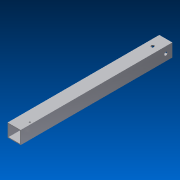
# Autodesk Inventor part: SwitchBarSupport
Saved by Autodesk Inventor 2013 (Build 170138000, 138)
## iProperties
Created: 2013-07-20
Part Number: SwitchBarSupport
Material: Aluminum 6061
Document SubType Name: Modeling
Designer: robotics
Density: 1 g/cm^3
Author: robotics
Autodesk Inventor part; units mm, degrees
ref_plane "YZ Plane" through (0, 0, 0) normal (1, 0, 0) x (0, 1, 0)
ref_plane "XZ Plane" through (0, 0, 0) normal (0, 1, 0) x (-1, 0, 0)
ref_plane "XY Plane" through (0, 0, 0) normal (0, 0, 1) x (1, 0, 0)
sketch "Sketch1" plane through (0, 0, 0) normal (0, 0, 1) x (1, 0, 0)
  line L0 (0, 0) -> (25.4, 0)
  line L1 (25.4, 0) -> (25.4, 25.4)
  line L2 (25.4, 25.4) -> (0, 25.4)
  line L3 (0, 25.4) -> (0, 0)
  line L4 (1.5875, 1.5875) -> (23.8125, 1.5875)
  line L5 (23.8125, 1.5875) -> (23.8125, 23.8125)
  line L6 (23.8125, 23.8125) -> (1.5875, 23.8125)
  line L7 (1.5875, 23.8125) -> (1.5875, 1.5875)
  dimension "d0" = 25.4
  dimension "d1" = 25.4
  dimension "d2" = 1.5875
  dimension "d3" = 1.5875
  dimension "d4" = 1.5875
  dimension "d5" = 1.5875
  constraints: 16 end point, 4 parallel, 2 horizontal, 2 perpendicular
  measures "d0" distance of L2.end L0.start
  measures "d1" distance of L1.end L2.end
  measures "d2" distance between parallel lines of L6 L2
  measures "d3" distance between parallel lines of L0 L4
  measures "d4" distance between parallel lines of L1 L5
  measures "d5" distance between parallel lines of L7 L3
extrude "Extrusion1" add sketch "Sketch1" along normal blind 294.894
sketch "Sketch2" plane through (0, 0, 0) normal (0, -1, 0) x (1, 0, 0)
  line L0 (0, 294.894) -> (25.4, 294.894) projected
  point P0 (21.1377, 272.796)
  dimension "d15" = 22.098
  measures "d15" distance from line of point (21.138, 272.796) L0
hole "Hole1" at (21.1377, 0, 272.796) direction (0, 1, 0) diameter 2.9972 end through all
sketch "Sketch3" plane through (0, 0, 0) normal (-1, 0, 0) x (0, 0, 1)
  line L0 (0, 25.4) -> (0, 0) projected
  line L1 (0, 25.4) -> (294.894, 25.4) projected
  point P0 (12.7, 12.7)
  dimension "d16" = 12.7
  dimension "d17" = 12.7
  measures "d16" distance from line of point (12.7, 12.7) L1
  measures "d17" distance from line of L0 point (12.7, 12.7)
hole "Hole2" at (0, 12.7, 12.7) direction (1, 0, 0) diameter 6.35 end through all
sketch "Sketch4" plane through (0, 0, 0) normal (0, -1, 0) x (1, 0, 0)
  line L0 (0, 0) -> (25.4, 0) projected
  line L1 (0, 0) -> (0, 294.894) projected
  point P0 (12.7, 25.4)
  dimension "d25" = 25.4
  dimension "d26" = 12.7
  measures "d25" distance from line of L0 point (12.7, 25.4)
  measures "d26" distance from line of L1 point (12.7, 25.4)
hole "Hole3" at (12.7, 0, 25.4) direction (0, 1, 0) diameter 6.35 end through all
body "Solid1"
